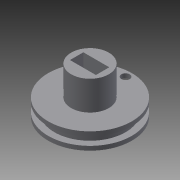
# Autodesk Inventor part: Stpper Wheel 2
Saved by Autodesk Inventor 2015 (Build 190159000, 159)
## iProperties
Created: 2016-05-27
Part Number: Stpper Wheel 2
Material: Generic
Document SubType Name: Modeling
Designer: Toby
Density: 1 g/cm^3
Appearance: Default
Author: Toby
Autodesk Inventor part; units mm, degrees
ref_plane "YZ Plane" through (0, 0, 0) normal (1, 0, 0) x (0, 1, 0)
ref_plane "XZ Plane" through (0, 0, 0) normal (0, 1, 0) x (-1, 0, 0)
ref_plane "XY Plane" through (0, 0, 0) normal (0, 0, 1) x (1, 0, 0)
sketch "Sketch1" plane through (0, 0, 0) normal (0, 0, 1) x (1, 0, 0)
  circle A0 centre (0, 0) radius 10
  circle A1 centre (0, 0) radius 8.5
  dimension "d0" = 20
  dimension "d1" = 17
  constraints: 2 centre point, 2 coincident
  measures "d0" diameter of A0
  measures "d1" diameter of A1
extrude "Extrusion1" add sketch "Sketch1" along normal blind 1 contours A0 | A1
sketch "Sketch2" plane through (0, 0, 1) normal (0, 0, 1) x (1, 0, 0)
  circle A0 centre (0, 0) radius 8.5
  dimension "d4" = 17
  constraints: 1 centre point, 1 coincident
  measures "d4" diameter of A0
extrude "Extrusion2" add sketch "Sketch2" along normal blind 2
sketch "Sketch3" plane through (0, 0, 3) normal (0, 0, 1) x (1, 0, 0)
  circle A0 centre (0, 0) radius 10
  constraints: 1 centre point, 1 coincident
extrude "Extrusion3" add sketch "Sketch3" along normal blind 1
sketch "Sketch4" plane through (0, 0, 4) normal (0, 0, 1) x (1, 0, 0)
  circle A0 centre (0, 0) radius 4.5
  line L0 (-3.1, 1.51) -> (3.1, 1.51)
  line L1 (3.1, 1.51) -> (3.1, -1.69)
  line L2 (3.1, -1.69) -> (-3.1, -1.69)
  line L3 (-3.1, -1.69) -> (-3.1, 1.51)
  dimension "d9" = 9
  dimension "d10" = 6.2
  dimension "d11" = 3.2
  dimension "d12" = 1.51
  dimension "d13" = 3.1
  constraints: 8 end point, 2 parallel, 1 centre point, 1 coincident, 1 horizontal, 1 perpendicular
  measures "d9" diameter of A0
  measures "d10" distance of L0.start L0.end
  measures "d11" distance of L2.end L0.start
  measures "d12" distance from line of point (0, 0) L0
  measures "d13" distance from line of point (0, 0) L1
extrude "Extrusion4" add sketch "Sketch4" along normal blind 7
sketch "Sketch5" plane through (0, 0, 4) normal (0, 0, 1) x (1, 0, 0)
  circle A0 centre (0, 0) radius 8.5 projected
  circle A1 centre (0, 8.5) radius 1
  dimension "d16" = 2
  constraints: 1 centre point, 1 vertical alignment, 1 other
  measures "d16" diameter of A1
extrude "Extrusion5" cut sketch "Sketch5" against normal blind 7 contours A1 A0 | A0 A1 picked at (0.0387, 8.1646) picked at (0.0312, 8.8275)
body "Solid1"
